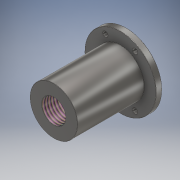
# Autodesk Inventor part: RNFBL2005A2.5S
Saved by Autodesk Inventor 2018 (Build 220112000, 112)
## iProperties
Created: 2018-04-10
Part Number: RNFBL2005A2.5S
Material: Steel, Carbon
Document SubType Name: Modeling
Designer: P136265
Density: 7.85 g/cm^3
Appearance: Semi-Polished
Author: P136265
Autodesk Inventor part; units mm, degrees
ref_plane "YZ Plane" through (0, 0, 0) normal (1, 0, 0) x (0, 1, 0)
ref_plane "XZ Plane" through (0, 0, 0) normal (0, 1, 0) x (-1, 0, 0)
ref_plane "XY Plane" through (0, 0, 0) normal (0, 0, 1) x (1, 0, 0)
sketch "Sketch1" plane through (0, 0, 0) normal (0, 1, 0) x (-1, 0, 0)
  circle A0 centre (0, 0) radius 30
  dimension "d0" = 60
  constraints: 1 centre point, 1 coincident
  measures "d0" diameter of A0
extrude "Extrusion1" add sketch "Sketch1" along normal blind 5
sketch "Sketch2" plane through (0, 0, 0) normal (0, -1, 0) x (1, 0, 0)
  circle A0 centre (0, 0) radius 20
  dimension "d3" = 40
  constraints: 1 centre point, 1 coincident
  measures "d3" diameter of A0
extrude "Extrusion2" add sketch "Sketch2" along normal blind 56
sketch "Sketch3" plane through (0, 5, 0) normal (0, 1, 0) x (1, 0, 0)
  circle A0 centre (0, 0) radius 2.5 construction
  dimension "d6" = 5
  constraints: 1 centre point, 1 coincident
  measures "d6" diameter of A0
hole "Hole1" at (0, 5, 0) direction (0, -1, 0) diameter 20 end through all
thread "Thread1" size "M20x2.5" class "6H" standard "ANSI Metric M Profile" full length
sketch "Sketch4" plane through (0, 5, 0) normal (0, 1, 0) x (1, 0, 0)
  line L0 (0, 0) -> (0, 50) construction
  line L1 (0, 0) -> (25, 43.3013) construction
  line L2 (0, 0) -> (-25, 43.3013) construction
  circle A0 centre (0, 0) radius 25 construction
  circle A1 centre (12.5, 21.6506) radius 2 construction
  circle A2 centre (-12.5, 21.6506) radius 2 construction
  line L3 (0, 0) -> (25, 0) construction
  circle A3 centre (12.5, -21.6506) radius 2 construction
  circle A4 centre (-12.5, -21.6506) radius 2 construction
  dimension "d16" = 50
  dimension "d17" = 50
  dimension "d18" = 30
  dimension "d19" = 50
  dimension "d20" = 4
  dimension "d21" = 4
  constraints: 8 end point, 5 centre point, 3 point on circle, 3 symmetric about line, 2 midpoint, 1 coincident, 1 horizontal, 1 vertical, 2 other
  measures "d16" distance of L0.start L0.end
  measures "d17" distance of L0.start L1.end
  measures "d18" angle of L0 L1
  measures "d19" diameter of A0
  measures "d20" diameter of A1
  measures "d21" diameter of A2
hole "Hole2" at (12.5, 5, -21.6506) at (-12.5, 5, -21.6506) at (12.5, 5, 21.6506) at (-12.5, 5, 21.6506) direction (0, -1, 0) diameter 4.5 end through all
fillet "Fillet1" radius 0.25 6 edges at (30, 0, 0) (30, 5, 0) (-20, -56, 0) (0, -56, -10) (-20, 0, 0) (0, 5, -10)
body "Solid1"
